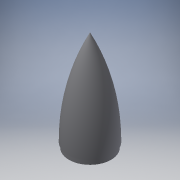
# Autodesk Inventor part: Nose Cone
Saved by Autodesk Inventor 2019.4 (Build 234330000, 330)
## iProperties
Created: 2022-01-22
Part Number: Nose Cone
Material: Generic
Document SubType Name: Modeling
Designer: juand
Density: 1 g/cm^3
Appearance: Default
Author: juand
Autodesk Inventor part; units mm, degrees
ref_plane "YZ Plane" through (0, 0, 0) normal (1, 0, 0) x (0, 1, 0)
ref_plane "XZ Plane" through (0, 0, 0) normal (0, 1, 0) x (-1, 0, 0)
ref_plane "XY Plane" through (0, 0, 0) normal (0, 0, 1) x (1, 0, 0)
sketch "Sketch1" plane through (0, 0, 0) normal (1, 0, 0) x (0, 1, 0)
  arc A0 (0, -32.5) -> (140, 0) centre (3.407, 270.6123) ccw
  line L0 (0, -32.5) -> (0, -31)
  line L1 (0, -31) -> (-7, -31)
  line L2 (-7, -31) -> (-7, -29.8)
  arc A1 (1.2, -31.3111) -> (137.3158, 0) centre (3.407, 270.6123) ccw
  line L3 (1.2, -31.3111) -> (1.2, -29.8)
  line L4 (1.2, -29.8) -> (-7, -29.8)
  line L5 (140, 0) -> (137.3158, 0)
  line L6 (-7, 0) -> (-5.8, 0)
  line L7 (178.1223, 0) -> (-98.5362, 0) construction
  point P0 (0, 0)
  dimension "d0" = 32.5
  dimension "d1" = 140
  dimension "d2" = 1.5
  dimension "d3" = 7
  dimension "d4" = 1.2
  constraints: 16 end point, 4 point on circle, 3 horizontal, 3 perpendicular, 2 centre point
  measures "d0" distance of point (0, 0) L0.start
  measures "d1" distance of point (0, 0) L5.start
  measures "d2" distance of L0.start L0.end
  measures "d3" distance of L0.end L1.end
  measures "d4" radial gap between concentric circles of A0 A1
revolve "Revolution1" add sketch "Sketch1" angle 360 about axis through (0, 178.1223, 0) along (0, -1, 0)
body "Solid1"
